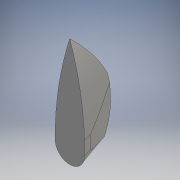
# Autodesk Inventor part: Part2
Saved by Autodesk Inventor 2016 (Build 200138000, 138)
## iProperties
Created: 2016-05-15
Part Number: Part2
Material: Generic
Document SubType Name: Modeling
Designer: Mauricio
Density: 1 g/cm^3
Appearance: Default
Author: Mauricio
Autodesk Inventor part; units mm, degrees
ref_plane "XZ Plane" through (0, 0, 0) normal (0, 1, 0) x (-1, 0, 0)
ref_plane "XY Plane" through (0, 0, 0) normal (0, 0, 1) x (1, 0, 0)
sketch "Sketch4" plane through (0, 0, 0) normal (0, 1, 0) x (-1, 0, 0)
  line L0 (-5800, -1270.133346) -> (-5792.28773, -1270.133346)
  line L1 (-5510.415149, -1125.340921) -> (-5510.415149, -1107.937911)
  line L2 (-5800, -991.627615) -> (-5800, -1125.340921)
  arc A0 (-5800, -1125.340921) -> (-5510.415149, -1125.340921) centre (-5655.207574, -1125.340921) ccw
  arc A1 (-5510.415149, -1125.340921) -> (-5655.207574, -197.261411) centre (-8501.403943, -1116.639416) ccw
  arc A2 (-5655.207574, -197.261411) -> (-5800, -1125.340921) centre (-3181.769662, -1058.484268) ccw
  line L3 (-5792.28773, -1270.133346) -> (-5510.415149, -1270.133346)
  line L4 (-5510.415149, -1270.133346) -> (-5510.415149, -1125.340921)
  line L5 (-5792.28773, -1125.340921) -> (-5792.28773, -1270.133346)
  point P0 (0, 0)
  point P1 (0, 0)
  constraints: 12 end point, 9 point on circle, 3 centre point, 3 tangent, 2 horizontal, 2 parallel, 2 perpendicular
extrude "Extrusion1" add sketch "Sketch4" along normal blind 400 draft -17 contours A0 L2 A2 A1 L1
ref_plane "Work Plane4" through (5800, 0, -1288.090921) normal (0, 0, 1) x (-0.2923717, 0.9563048, 0)
ref_plane "Work Plane3" through (5800, 0, -1125.340921) normal (0, 0, 1) x (-0.2923717, 0.9563048, 0)
sketch "Sketch5" plane through (5800, 0, -1288.090921) normal (0, 0, 1) x (-0.2923717, 0.9563048, 0)
  line L0 (0, 0) -> (84.666417, 276.931371)
  line L1 (42.333208, 144.792426) -> (424.082291, 144.792426)
  ellipse E0 centre (42.333208, 138.465685) end of major axis (794.143281, 138.465685) minor radius 138.685721 (0, 0) -> (84.666417, 276.931371) ccw
  line L2 (0, 0) -> (0, 276.931371)
  point P0 (1695.755887, 5546.567585)
  point P1 (424.082291, 18.989223)
  constraints: 2 end point, 1 horizontal, 1 midpoint, 1 vertical, 5 other
extrude "Extrusion2" cut sketch "Sketch5" along normal blind 1274.25 keep common part
ref_plane "Work Plane5" through (5851, 0, 0) normal (1, 0, 0) x (0, 1, 0)
sketch "Sketch6" plane through (5851, 0, 0) normal (1, 0, 0) x (0, 1, 0)
  line L0 (0, -1270.133346) -> (0, -1125.340921)
  line L1 (0, -1270.133346) -> (0, -992.638575)
  line L2 (0, -1107.937911) -> (0, -197.261411)
  line L3 (0, -992.638575) -> (0, -197.261411)
  line L4 (0, -992.638575) -> (400, -992.638575)
  line L5 (0, -197.261411) -> (0, -197.261411)
  line L6 (0, -197.261411) -> (400, -197.261411)
  ellipse E0 centre (0, -991.627615) end of major axis (0, -197.261411) minor radius 400.000324 (396.639434, -888.868932) -> (0, -197.261411) ccw
  ellipse E1 centre (0, -922.168604) end of major axis (398.468254, -922.168604) minor radius 347.964742 (0, -1270.133346) -> (396.639434, -888.868932) ccw
  point P0 (0, 0)
  dimension "d9" = 400
  constraints: 7 end point, 2 horizontal, 2 point on line, 2 vertical, 11 other
  measures "d9" distance of L1.end L4.end
extrude "Extrusion3" cut sketch "Sketch6" against normal blind 1274.25 keep common part
body "Solid1"
